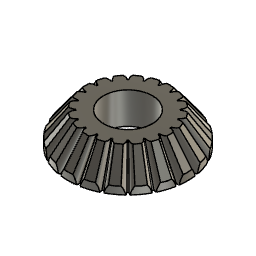
Bevel Gear (Autodesk Fusion 360 design; units mm, degrees)
Autodesk Fusion 360 part; units mm, degrees
sketch "Base" plane through (0, 0, 0) normal (0, 0, 1) x (1, 0, 0)
  line L0 (3, 40) -> (-3, 40)
  arc A0 (4.9465, 34.6487) -> (3, 40) centre (-1.791, 35.2276) ccw
  arc A1 (-3, 40) -> (-4.9465, 34.6487) centre (1.791, 35.2276) ccw
  line L1 (-9.5075, 38.9693) -> (-15.2138, 37.1152)
  arc A2 (-6.0026, 34.4814) -> (-9.5075, 38.9693) centre (-12.5893, 32.95) ccw
  arc A3 (-15.2138, 37.1152) -> (-15.4114, 31.4243) centre (-9.1826, 34.0569) ccw
  line L2 (-21.0844, 34.124) -> (-25.9385, 30.5973)
  arc A4 (-16.3642, 30.9389) -> (-21.0844, 34.124) centre (-22.1552, 27.447) ccw
  arc A5 (-25.9385, 30.5973) -> (-24.3678, 25.1239) centre (-19.2574, 29.5525) ccw
  line L3 (-30.5973, 25.9385) -> (-34.124, 21.0844)
  arc A6 (-25.1239, 24.3678) -> (-30.5973, 25.9385) centre (-29.5525, 19.2574) ccw
  arc A7 (-34.124, 21.0844) -> (-30.9389, 16.3642) centre (-27.447, 22.1552) ccw
  line L4 (-37.1152, 15.2138) -> (-38.9693, 9.5075)
  arc A8 (-31.4243, 15.4114) -> (-37.1152, 15.2138) centre (-34.0569, 9.1826) ccw
  arc A9 (-38.9693, 9.5075) -> (-34.4814, 6.0026) centre (-32.95, 12.5893) ccw
  line L5 (-40, 3) -> (-40, -3)
  arc A10 (-34.6487, 4.9465) -> (-40, 3) centre (-35.2276, -1.791) ccw
  arc A11 (-40, -3) -> (-34.6487, -4.9465) centre (-35.2276, 1.791) ccw
  line L6 (-38.9693, -9.5075) -> (-37.1152, -15.2138)
  arc A12 (-34.4814, -6.0026) -> (-38.9693, -9.5075) centre (-32.95, -12.5893) ccw
  arc A13 (-37.1152, -15.2138) -> (-31.4243, -15.4114) centre (-34.0569, -9.1826) ccw
  line L7 (-34.124, -21.0844) -> (-30.5973, -25.9385)
  arc A14 (-30.9389, -16.3642) -> (-34.124, -21.0844) centre (-27.447, -22.1552) ccw
  arc A15 (-30.5973, -25.9385) -> (-25.1239, -24.3678) centre (-29.5525, -19.2574) ccw
  line L8 (-25.9385, -30.5973) -> (-21.0844, -34.124)
  arc A16 (-24.3678, -25.1239) -> (-25.9385, -30.5973) centre (-19.2574, -29.5525) ccw
  arc A17 (-21.0844, -34.124) -> (-16.3642, -30.9389) centre (-22.1552, -27.447) ccw
  line L9 (-15.2138, -37.1152) -> (-9.5075, -38.9693)
  arc A18 (-15.4114, -31.4243) -> (-15.2138, -37.1152) centre (-9.1826, -34.0569) ccw
  arc A19 (-9.5075, -38.9693) -> (-6.0026, -34.4814) centre (-12.5893, -32.95) ccw
  line L10 (-3, -40) -> (3, -40)
  arc A20 (-4.9465, -34.6487) -> (-3, -40) centre (1.791, -35.2276) ccw
  arc A21 (3, -40) -> (4.9465, -34.6487) centre (-1.791, -35.2276) ccw
  line L11 (9.5075, -38.9693) -> (15.2138, -37.1152)
  arc A22 (6.0026, -34.4814) -> (9.5075, -38.9693) centre (12.5893, -32.95) ccw
  arc A23 (15.2138, -37.1152) -> (15.4114, -31.4243) centre (9.1826, -34.0569) ccw
  line L12 (21.0844, -34.124) -> (25.9385, -30.5973)
  arc A24 (16.3642, -30.9389) -> (21.0844, -34.124) centre (22.1552, -27.447) ccw
  arc A25 (25.9385, -30.5973) -> (24.3678, -25.1239) centre (19.2574, -29.5525) ccw
  line L13 (30.5973, -25.9385) -> (34.124, -21.0844)
  arc A26 (25.1239, -24.3678) -> (30.5973, -25.9385) centre (29.5525, -19.2574) ccw
  arc A27 (34.124, -21.0844) -> (30.9389, -16.3642) centre (27.447, -22.1552) ccw
  line L14 (37.1152, -15.2138) -> (38.9693, -9.5075)
  arc A28 (31.4243, -15.4114) -> (37.1152, -15.2138) centre (34.0569, -9.1826) ccw
  arc A29 (38.9693, -9.5075) -> (34.4814, -6.0026) centre (32.95, -12.5893) ccw
  line L15 (40, -3) -> (40, 3)
  arc A30 (34.6487, -4.9465) -> (40, -3) centre (35.2276, 1.791) ccw
  arc A31 (40, 3) -> (34.6487, 4.9465) centre (35.2276, -1.791) ccw
  line L16 (38.9693, 9.5075) -> (37.1152, 15.2138)
  arc A32 (34.4814, 6.0026) -> (38.9693, 9.5075) centre (32.95, 12.5893) ccw
  arc A33 (37.1152, 15.2138) -> (31.4243, 15.4114) centre (34.0569, 9.1826) ccw
  line L17 (34.124, 21.0844) -> (30.5973, 25.9385)
  arc A34 (30.9389, 16.3642) -> (34.124, 21.0844) centre (27.447, 22.1552) ccw
  arc A35 (30.5973, 25.9385) -> (25.1239, 24.3678) centre (29.5525, 19.2574) ccw
  line L18 (25.9385, 30.5973) -> (21.0844, 34.124)
  arc A36 (24.3678, 25.1239) -> (25.9385, 30.5973) centre (19.2574, 29.5525) ccw
  arc A37 (21.0844, 34.124) -> (16.3642, 30.9389) centre (22.1552, 27.447) ccw
  line L19 (15.2138, 37.1152) -> (9.5075, 38.9693)
  arc A38 (15.4114, 31.4243) -> (15.2138, 37.1152) centre (9.1826, 34.0569) ccw
  arc A39 (9.5075, 38.9693) -> (6.0026, 34.4814) centre (12.5893, 32.95) ccw
  arc A40 (-4.9465, 34.6487) -> (-6.0026, 34.4814) centre (0, 0) ccw
  arc A41 (-15.4114, 31.4243) -> (-16.3642, 30.9389) centre (0, 0) ccw
  arc A42 (-24.3678, 25.1239) -> (-25.1239, 24.3678) centre (0, 0) ccw
  arc A43 (-30.9389, 16.3642) -> (-31.4243, 15.4114) centre (0, 0) ccw
  arc A44 (-34.4814, 6.0026) -> (-34.6487, 4.9465) centre (0, 0) ccw
  arc A45 (-34.6487, -4.9465) -> (-34.4814, -6.0026) centre (0, 0) ccw
  arc A46 (-31.4243, -15.4114) -> (-30.9389, -16.3642) centre (0, 0) ccw
  arc A47 (-25.1239, -24.3678) -> (-24.3678, -25.1239) centre (0, 0) ccw
  arc A48 (-16.3642, -30.9389) -> (-15.4114, -31.4243) centre (0, 0) ccw
  arc A49 (-6.0026, -34.4814) -> (-4.9465, -34.6487) centre (0, 0) ccw
  arc A50 (4.9465, -34.6487) -> (6.0026, -34.4814) centre (0, 0) ccw
  arc A51 (15.4114, -31.4243) -> (16.3642, -30.9389) centre (0, 0) ccw
  arc A52 (24.3678, -25.1239) -> (25.1239, -24.3678) centre (0, 0) ccw
  arc A53 (30.9389, -16.3642) -> (31.4243, -15.4114) centre (0, 0) ccw
  arc A54 (34.4814, -6.0026) -> (34.6487, -4.9465) centre (0, 0) ccw
  arc A55 (34.6487, 4.9465) -> (34.4814, 6.0026) centre (0, 0) ccw
  arc A56 (31.4243, 15.4114) -> (30.9389, 16.3642) centre (0, 0) ccw
  arc A57 (25.1239, 24.3678) -> (24.3678, 25.1239) centre (0, 0) ccw
  arc A58 (16.3642, 30.9389) -> (15.4114, 31.4243) centre (0, 0) ccw
  arc A59 (6.0026, 34.4814) -> (4.9465, 34.6487) centre (0, 0) ccw
  line L20 (1.95, 26, 19.5) -> (-1.95, 26, 19.5)
  line L21 (6.1799, -25.3301, 19.5) -> (9.889, -24.1249, 19.5)
  line L22 (-26, 1.95, 19.5) -> (-26, -1.95, 19.5)
  line L23 (26, -1.95, 19.5) -> (26, 1.95, 19.5)
  line L24 (-16.86, -19.8883, 19.5) -> (-13.7048, -22.1806, 19.5)
  arc A60 through (-16.3305, -15.8391, 19.5) (-16.0867, -16.0867, 19.5) (-15.8391, -16.3305, 19.5)
  arc A61 through (9.889, -24.1249, 19.5) (10.3616, -22.2895, 19.5) (10.0174, -20.4258, 19.5)
  line L25 (24.1249, -9.889, 19.5) -> (25.3301, -6.1799, 19.5)
  arc A62 through (-20.4258, 10.0174, 19.5) (-22.2895, 10.3616, 19.5) (-24.1249, 9.889, 19.5)
  arc A63 through (-9.889, 24.1249, 19.5) (-10.3616, 22.2895, 19.5) (-10.0174, 20.4258, 19.5)
  line L26 (-19.8883, 16.86, 19.5) -> (-22.1806, 13.7048, 19.5)
  arc A64 through (22.5217, -3.2152, 19.5) (24.4005, -2.9666, 19.5) (26, -1.95, 19.5)
  arc A65 through (1.95, -26, 19.5) (2.9666, -24.4005, 19.5) (3.2152, -22.5217, 19.5)
  arc A66 through (3.9017, -22.4129, 19.5) (4.7188, -24.123, 19.5) (6.1799, -25.3301, 19.5)
  arc A67 through (16.3305, -15.8391, 19.5) (17.9967, -16.7423, 19.5) (19.8883, -16.86, 19.5)
  arc A68 through (-10.6367, 20.1103, 19.5) (-11.9422, 21.4841, 19.5) (-13.7048, 22.1806, 19.5)
  line L27 (-24.1249, 9.889, 19.5) -> (-25.3301, 6.1799, 19.5)
  arc A69 through (-24.1249, -9.889, 19.5) (-22.2895, -10.3616, 19.5) (-20.4258, -10.0174, 19.5)
  arc A70 through (-16.3305, 15.8391, 19.5) (-17.9967, 16.7423, 19.5) (-19.8883, 16.86, 19.5)
  arc A71 through (-26, -1.95, 19.5) (-24.4005, -2.9666, 19.5) (-22.5217, -3.2152, 19.5)
  arc A72 through (15.8391, 16.3305, 19.5) (16.7423, 17.9967, 19.5) (16.86, 19.8883, 19.5)
  arc A73 through (-20.4258, -10.0174, 19.5) (-20.2704, -10.3283, 19.5) (-20.1103, -10.6367, 19.5)
  line L28 (-9.889, -24.1249, 19.5) -> (-6.1799, -25.3301, 19.5)
  arc A74 through (24.1249, 9.889, 19.5) (22.2895, 10.3616, 19.5) (20.4258, 10.0174, 19.5)
  line L29 (-22.1806, -13.7048, 19.5) -> (-19.8883, -16.86, 19.5)
  arc A75 through (16.3305, 15.8391, 19.5) (16.0867, 16.0867, 19.5) (15.8391, 16.3305, 19.5)
  line L30 (19.8883, -16.86, 19.5) -> (22.1806, -13.7048, 19.5)
  line L31 (9.889, 24.1249, 19.5) -> (6.1799, 25.3301, 19.5)
  arc A76 through (-15.8391, -16.3305, 19.5) (-16.7423, -17.9967, 19.5) (-16.86, -19.8883, 19.5)
  arc A77 through (-15.8391, 16.3305, 19.5) (-16.0867, 16.0867, 19.5) (-16.3305, 15.8391, 19.5)
  arc A78 through (-22.5217, -3.2152, 19.5) (-22.4699, -3.5589, 19.5) (-22.4129, -3.9017, 19.5)
  arc A79 through (25.3301, -6.1799, 19.5) (24.123, -4.7188, 19.5) (22.4129, -3.9017, 19.5)
  line L32 (-13.7048, 22.1806, 19.5) -> (-16.86, 19.8883, 19.5)
  arc A80 through (22.1806, -13.7048, 19.5) (21.4841, -11.9422, 19.5) (20.1103, -10.6367, 19.5)
  arc A81 through (3.2152, -22.5217, 19.5) (3.5589, -22.4699, 19.5) (3.9017, -22.4129, 19.5)
  arc A82 through (-22.1806, 13.7048, 19.5) (-21.4841, 11.9422, 19.5) (-20.1103, 10.6367, 19.5)
  arc A83 through (22.4129, -3.9017, 19.5) (22.4699, -3.5589, 19.5) (22.5217, -3.2152, 19.5)
  arc A84 through (-10.0174, 20.4258, 19.5) (-10.3283, 20.2704, 19.5) (-10.6367, 20.1103, 19.5)
  arc A85 through (-3.2152, 22.5217, 19.5) (-3.5589, 22.4699, 19.5) (-3.9017, 22.4129, 19.5)
  arc A86 through (-1.95, 26, 19.5) (-2.9666, 24.4005, 19.5) (-3.2152, 22.5217, 19.5)
  arc A87 through (-22.4129, 3.9017, 19.5) (-22.4699, 3.5589, 19.5) (-22.5217, 3.2152, 19.5)
  arc A88 through (-16.86, 19.8883, 19.5) (-16.7423, 17.9967, 19.5) (-15.8391, 16.3305, 19.5)
  arc A89 through (-3.9017, 22.4129, 19.5) (-4.7188, 24.123, 19.5) (-6.1799, 25.3301, 19.5)
  arc A90 through (-25.3301, 6.1799, 19.5) (-24.123, 4.7188, 19.5) (-22.4129, 3.9017, 19.5)
  arc A91 through (-22.5217, 3.2152, 19.5) (-24.4005, 2.9666, 19.5) (-26, 1.95, 19.5)
  arc A92 through (-10.6367, -20.1103, 19.5) (-10.3283, -20.2704, 19.5) (-10.0174, -20.4258, 19.5)
  arc A93 through (-20.1103, 10.6367, 19.5) (-20.2704, 10.3283, 19.5) (-20.4258, 10.0174, 19.5)
  arc A94 through (-20.1103, -10.6367, 19.5) (-21.4841, -11.9422, 19.5) (-22.1806, -13.7048, 19.5)
  arc A95 through (20.1103, 10.6367, 19.5) (21.4841, 11.9422, 19.5) (22.1806, 13.7048, 19.5)
  arc A96 through (3.9017, 22.4129, 19.5) (3.5589, 22.4699, 19.5) (3.2152, 22.5217, 19.5)
  arc A97 through (22.4129, 3.9017, 19.5) (24.123, 4.7188, 19.5) (25.3301, 6.1799, 19.5)
  arc A98 through (3.2152, 22.5217, 19.5) (2.9666, 24.4005, 19.5) (1.95, 26, 19.5)
  arc A99 through (-19.8883, -16.86, 19.5) (-17.9967, -16.7423, 19.5) (-16.3305, -15.8391, 19.5)
  arc A100 through (10.0174, -20.4258, 19.5) (10.3283, -20.2704, 19.5) (10.6367, -20.1103, 19.5)
  arc A101 through (10.6367, 20.1103, 19.5) (10.3283, 20.2704, 19.5) (10.0174, 20.4258, 19.5)
  arc A102 through (15.8391, -16.3305, 19.5) (16.0867, -16.0867, 19.5) (16.3305, -15.8391, 19.5)
  arc A103 through (13.7048, 22.1806, 19.5) (11.9422, 21.4841, 19.5) (10.6367, 20.1103, 19.5)
  arc A104 through (10.6367, -20.1103, 19.5) (11.9422, -21.4841, 19.5) (13.7048, -22.1806, 19.5)
  arc A105 through (20.4258, -10.0174, 19.5) (22.2895, -10.3616, 19.5) (24.1249, -9.889, 19.5)
  arc A106 through (-3.9017, -22.4129, 19.5) (-3.5589, -22.4699, 19.5) (-3.2152, -22.5217, 19.5)
  line L33 (16.86, 19.8883, 19.5) -> (13.7048, 22.1806, 19.5)
  arc A107 through (16.86, -19.8883, 19.5) (16.7423, -17.9967, 19.5) (15.8391, -16.3305, 19.5)
  arc A108 through (26, 1.95, 19.5) (24.4005, 2.9666, 19.5) (22.5217, 3.2152, 19.5)
  line L34 (22.1806, 13.7048, 19.5) -> (19.8883, 16.86, 19.5)
  arc A109 through (6.1799, 25.3301, 19.5) (4.7188, 24.123, 19.5) (3.9017, 22.4129, 19.5)
  arc A110 through (19.8883, 16.86, 19.5) (17.9967, 16.7423, 19.5) (16.3305, 15.8391, 19.5)
  arc A111 through (-6.1799, -25.3301, 19.5) (-4.7188, -24.123, 19.5) (-3.9017, -22.4129, 19.5)
  arc A112 through (10.0174, 20.4258, 19.5) (10.3616, 22.2895, 19.5) (9.889, 24.1249, 19.5)
  arc A113 through (-10.0174, -20.4258, 19.5) (-10.3616, -22.2895, 19.5) (-9.889, -24.1249, 19.5)
  arc A114 through (-3.2152, -22.5217, 19.5) (-2.9666, -24.4005, 19.5) (-1.95, -26, 19.5)
  arc A115 through (22.5217, 3.2152, 19.5) (22.4699, 3.5589, 19.5) (22.4129, 3.9017, 19.5)
  arc A116 through (20.4258, 10.0174, 19.5) (20.2704, 10.3283, 19.5) (20.1103, 10.6367, 19.5)
  line L35 (-25.3301, -6.1799, 19.5) -> (-24.1249, -9.889, 19.5)
  line L36 (25.3301, 6.1799, 19.5) -> (24.1249, 9.889, 19.5)
  arc A117 through (20.1103, -10.6367, 19.5) (20.2704, -10.3283, 19.5) (20.4258, -10.0174, 19.5)
  arc A118 through (-22.4129, -3.9017, 19.5) (-24.123, -4.7188, 19.5) (-25.3301, -6.1799, 19.5)
  line L37 (13.7048, -22.1806, 19.5) -> (16.86, -19.8883, 19.5)
  line L38 (-1.95, -26, 19.5) -> (1.95, -26, 19.5)
  arc A119 through (-13.7048, -22.1806, 19.5) (-11.9422, -21.4841, 19.5) (-10.6367, -20.1103, 19.5)
  line L39 (-6.1799, 25.3301, 19.5) -> (-9.889, 24.1249, 19.5)
  dimension "d7" = 360
  constraint coincident A40.centre A41.centre
  constraint concentric A40 A41
  constraint concentric A41 A42
  constraint concentric A42 A43
  constraint concentric A43 A44
  constraint concentric A44 A45
  constraint concentric A45 A46
  constraint concentric A46 A47
  constraint concentric A47 A48
  constraint concentric A48 A49
  constraint concentric A49 A50
  constraint concentric A50 A51
  constraint concentric A51 A52
  constraint concentric A52 A53
  constraint concentric A53 A54
  constraint concentric A54 A55
  constraint concentric A55 A56
  constraint concentric A56 A57
  constraint concentric A57 A58
  constraint concentric A58 A59
loft "Loft1" add profiles "Base", "Base" section 1 contours L20 L21 L22 L23 L24 A60 A61 L25 A62 A63 L26 A64 A65 A66 A67 A68 L27 A69 A70 A71 A72 A73 L28 A74 L29 A75 L30 L31 A76 A77 A78 A79 L32 A80 A81 A82 A83 A84 A85 A86 A87 A88 A89 A90 A91 A92 A93 A94 A95 A96 A97 A98 A99 A100 A101 A102 A103 A104 A105 A106 L33 A107 A108 L34 A109 A110 A111 A112 A113 A114 A115 A116 L35 L36 A117 A118 L37 L38 A119 L39 in plane through (0, 0, 19.5) normal (0, 0, 1) section 2
sketch "Cut" plane through (0, 0, 0) normal (0, 0, -1) x (1, 0, 0)
  line L0 (-15.2138, -37.1152) -> (-9.5075, -38.9693)
  arc A0 (-9.5075, -38.9693) -> (-6.0026, -34.4814) centre (-12.5893, -32.95) ccw
  arc A1 (-6.0026, -34.4814) -> (-4.9465, -34.6487) centre (0, 0) ccw
  arc A2 (-4.9465, -34.6487) -> (-3, -40) centre (1.791, -35.2276) ccw
  line L1 (-3, -40) -> (3, -40)
  arc A3 (3, -40) -> (4.9465, -34.6487) centre (-1.791, -35.2276) ccw
  arc A4 (4.9465, -34.6487) -> (6.0026, -34.4814) centre (0, 0) ccw
  arc A5 (6.0026, -34.4814) -> (9.5075, -38.9693) centre (12.5893, -32.95) ccw
  line L2 (9.5075, -38.9693) -> (15.2138, -37.1152)
  arc A6 (15.2138, -37.1152) -> (15.4114, -31.4243) centre (9.1826, -34.0569) ccw
  arc A7 (15.4114, -31.4243) -> (16.3642, -30.9389) centre (0, 0) ccw
  arc A8 (16.3642, -30.9389) -> (21.0844, -34.124) centre (22.1552, -27.447) ccw
  line L3 (21.0844, -34.124) -> (25.9385, -30.5973)
  arc A9 (25.9385, -30.5973) -> (24.3678, -25.1239) centre (19.2574, -29.5525) ccw
  arc A10 (24.3678, -25.1239) -> (25.1239, -24.3678) centre (0, 0) ccw
  arc A11 (25.1239, -24.3678) -> (30.5973, -25.9385) centre (29.5525, -19.2574) ccw
  line L4 (30.5973, -25.9385) -> (34.124, -21.0844)
  arc A12 (34.124, -21.0844) -> (30.9389, -16.3642) centre (27.447, -22.1552) ccw
  arc A13 (30.9389, -16.3642) -> (31.4243, -15.4114) centre (0, 0) ccw
  arc A14 (31.4243, -15.4114) -> (37.1152, -15.2138) centre (34.0569, -9.1826) ccw
  line L5 (37.1152, -15.2138) -> (38.9693, -9.5075)
  arc A15 (38.9693, -9.5075) -> (34.4814, -6.0026) centre (32.95, -12.5893) ccw
  arc A16 (34.4814, -6.0026) -> (34.6487, -4.9465) centre (0, 0) ccw
  arc A17 (34.6487, -4.9465) -> (40, -3) centre (35.2276, 1.791) ccw
  line L6 (40, -3) -> (40, 3)
  arc A18 (40, 3) -> (34.6487, 4.9465) centre (35.2276, -1.791) ccw
  arc A19 (34.6487, 4.9465) -> (34.4814, 6.0026) centre (0, 0) ccw
  arc A20 (34.4814, 6.0026) -> (38.9693, 9.5075) centre (32.95, 12.5893) ccw
  line L7 (38.9693, 9.5075) -> (37.1152, 15.2138)
  arc A21 (37.1152, 15.2138) -> (31.4243, 15.4114) centre (34.0569, 9.1826) ccw
  arc A22 (31.4243, 15.4114) -> (30.9389, 16.3642) centre (0, 0) ccw
  arc A23 (30.9389, 16.3642) -> (34.124, 21.0844) centre (27.447, 22.1552) ccw
  line L8 (34.124, 21.0844) -> (30.5973, 25.9385)
  arc A24 (30.5973, 25.9385) -> (25.1239, 24.3678) centre (29.5525, 19.2574) ccw
  arc A25 (25.1239, 24.3678) -> (24.3678, 25.1239) centre (0, 0) ccw
  arc A26 (24.3678, 25.1239) -> (25.9385, 30.5973) centre (19.2574, 29.5525) ccw
  line L9 (25.9385, 30.5973) -> (21.0844, 34.124)
  arc A27 (21.0844, 34.124) -> (16.3642, 30.9389) centre (22.1552, 27.447) ccw
  arc A28 (16.3642, 30.9389) -> (15.4114, 31.4243) centre (0, 0) ccw
  arc A29 (15.4114, 31.4243) -> (15.2138, 37.1152) centre (9.1826, 34.0569) ccw
  line L10 (15.2138, 37.1152) -> (9.5075, 38.9693)
  arc A30 (9.5075, 38.9693) -> (6.0026, 34.4814) centre (12.5893, 32.95) ccw
  arc A31 (6.0026, 34.4814) -> (4.9465, 34.6487) centre (0, 0) ccw
  arc A32 (4.9465, 34.6487) -> (3, 40) centre (-1.791, 35.2276) ccw
  line L11 (3, 40) -> (-3, 40)
  arc A33 (-3, 40) -> (-4.9465, 34.6487) centre (1.791, 35.2276) ccw
  arc A34 (-4.9465, 34.6487) -> (-6.0026, 34.4814) centre (0, 0) ccw
  arc A35 (-6.0026, 34.4814) -> (-9.5075, 38.9693) centre (-12.5893, 32.95) ccw
  line L12 (-9.5075, 38.9693) -> (-15.2138, 37.1152)
  arc A36 (-15.2138, 37.1152) -> (-15.4114, 31.4243) centre (-9.1826, 34.0569) ccw
  arc A37 (-15.4114, 31.4243) -> (-16.3642, 30.9389) centre (0, 0) ccw
  arc A38 (-16.3642, 30.9389) -> (-21.0844, 34.124) centre (-22.1552, 27.447) ccw
  line L13 (-21.0844, 34.124) -> (-25.9385, 30.5973)
  arc A39 (-25.9385, 30.5973) -> (-24.3678, 25.1239) centre (-19.2574, 29.5525) ccw
  arc A40 (-24.3678, 25.1239) -> (-25.1239, 24.3678) centre (0, 0) ccw
  arc A41 (-25.1239, 24.3678) -> (-30.5973, 25.9385) centre (-29.5525, 19.2574) ccw
  line L14 (-30.5973, 25.9385) -> (-34.124, 21.0844)
  arc A42 (-34.124, 21.0844) -> (-30.9389, 16.3642) centre (-27.447, 22.1552) ccw
  arc A43 (-30.9389, 16.3642) -> (-31.4243, 15.4114) centre (0, 0) ccw
  arc A44 (-31.4243, 15.4114) -> (-37.1152, 15.2138) centre (-34.0569, 9.1826) ccw
  line L15 (-37.1152, 15.2138) -> (-38.9693, 9.5075)
  arc A45 (-38.9693, 9.5075) -> (-34.4814, 6.0026) centre (-32.95, 12.5893) ccw
  arc A46 (-34.4814, 6.0026) -> (-34.6487, 4.9465) centre (0, 0) ccw
  arc A47 (-34.6487, 4.9465) -> (-40, 3) centre (-35.2276, -1.791) ccw
  line L16 (-40, 3) -> (-40, -3)
  arc A48 (-40, -3) -> (-34.6487, -4.9465) centre (-35.2276, 1.791) ccw
  arc A49 (-34.6487, -4.9465) -> (-34.4814, -6.0026) centre (0, 0) ccw
  arc A50 (-34.4814, -6.0026) -> (-38.9693, -9.5075) centre (-32.95, -12.5893) ccw
  line L17 (-38.9693, -9.5075) -> (-37.1152, -15.2138)
  arc A51 (-37.1152, -15.2138) -> (-31.4243, -15.4114) centre (-34.0569, -9.1826) ccw
  arc A52 (-31.4243, -15.4114) -> (-30.9389, -16.3642) centre (0, 0) ccw
  arc A53 (-30.9389, -16.3642) -> (-34.124, -21.0844) centre (-27.447, -22.1552) ccw
  line L18 (-34.124, -21.0844) -> (-30.5973, -25.9385)
  arc A54 (-30.5973, -25.9385) -> (-25.1239, -24.3678) centre (-29.5525, -19.2574) ccw
  arc A55 (-25.1239, -24.3678) -> (-24.3678, -25.1239) centre (0, 0) ccw
  arc A56 (-24.3678, -25.1239) -> (-25.9385, -30.5973) centre (-19.2574, -29.5525) ccw
  line L19 (-25.9385, -30.5973) -> (-21.0844, -34.124)
  arc A57 (-21.0844, -34.124) -> (-16.3642, -30.9389) centre (-22.1552, -27.447) ccw
  arc A58 (-16.3642, -30.9389) -> (-15.4114, -31.4243) centre (0, 0) ccw
  arc A59 (-15.4114, -31.4243) -> (-15.2138, -37.1152) centre (-9.1826, -34.0569) ccw
  circle A60 centre (0, 0) radius 36.7638
  circle A61 centre (0, 0) radius 43.0116
  constraint concentric A1 A60
  constraint concentric A60 A61
extrude "Extrude1" cut sketch "Cut" against normal blind 10 contours L0 A0 A59 A60 | A56 L19 A57 A60 | A2 L1 A3 A60 | A53 L18 A54 A60 | A5 L2 A6 A60 | A50 L17 A51 A60 | A8 L3 A9 A60 | A47 L16 A48 A60 | A11 L4 A12 A60 | A44 L15 A45 A60 | A14 L5 A15 A60 | A41 L14 A42 A60 | A17 L6 A18 A60 | A38 L13 A39 A60 | A20 L7 A21 A60 | A35 L12 A36 A60 | A23 L8 A24 A60 | A32 L11 A33 A60 | A26 L9 A27 A60 | A29 L10 A30 A60 | A61
sketch "Hole" plane through (0, 0, 19.5) normal (0, 0, 1) x (-1, 0, 0)
  line L0 (6.1799, -25.3301) -> (9.889, -24.1249)
  arc A0 (9.889, -24.1249) -> (10.0174, -20.4258) centre (5.9687, -22.137) ccw
  arc A1 (10.0174, -20.4258) -> (10.6367, -20.1103) centre (0, 0) ccw
  arc A2 (10.6367, -20.1103) -> (13.7048, -22.1806) centre (14.4009, -17.8406) ccw
  line L1 (13.7048, -22.1806) -> (16.86, -19.8883)
  arc A3 (16.86, -19.8883) -> (15.8391, -16.3305) centre (12.5173, -19.2091) ccw
  arc A4 (15.8391, -16.3305) -> (16.3305, -15.8391) centre (0, 0) ccw
  arc A5 (16.3305, -15.8391) -> (19.8883, -16.86) centre (19.2091, -12.5173) ccw
  line L2 (19.8883, -16.86) -> (22.1806, -13.7048)
  arc A6 (22.1806, -13.7048) -> (20.1103, -10.6367) centre (17.8406, -14.4009) ccw
  arc A7 (20.1103, -10.6367) -> (20.4258, -10.0174) centre (0, 0) ccw
  arc A8 (20.4258, -10.0174) -> (24.1249, -9.889) centre (22.137, -5.9687) ccw
  line L3 (24.1249, -9.889) -> (25.3301, -6.1799)
  arc A9 (25.3301, -6.1799) -> (22.4129, -3.9017) centre (21.4175, -8.183) ccw
  arc A10 (22.4129, -3.9017) -> (22.5217, -3.2152) centre (0, 0) ccw
  arc A11 (22.5217, -3.2152) -> (26, -1.95) centre (22.898, 1.1641) ccw
  line L4 (26, -1.95) -> (26, 1.95)
  arc A12 (26, 1.95) -> (22.5217, 3.2152) centre (22.898, -1.1641) ccw
  arc A13 (22.5217, 3.2152) -> (22.4129, 3.9017) centre (0, 0) ccw
  arc A14 (22.4129, 3.9017) -> (25.3301, 6.1799) centre (21.4175, 8.183) ccw
  line L5 (25.3301, 6.1799) -> (24.1249, 9.889)
  arc A15 (24.1249, 9.889) -> (20.4258, 10.0174) centre (22.137, 5.9687) ccw
  arc A16 (20.4258, 10.0174) -> (20.1103, 10.6367) centre (0, 0) ccw
  arc A17 (20.1103, 10.6367) -> (22.1806, 13.7048) centre (17.8406, 14.4009) ccw
  line L6 (22.1806, 13.7048) -> (19.8883, 16.86)
  arc A18 (19.8883, 16.86) -> (16.3305, 15.8391) centre (19.2091, 12.5173) ccw
  arc A19 (16.3305, 15.8391) -> (15.8391, 16.3305) centre (0, 0) ccw
  arc A20 (15.8391, 16.3305) -> (16.86, 19.8883) centre (12.5173, 19.2091) ccw
  line L7 (16.86, 19.8883) -> (13.7048, 22.1806)
  arc A21 (13.7048, 22.1806) -> (10.6367, 20.1103) centre (14.4009, 17.8406) ccw
  arc A22 (10.6367, 20.1103) -> (10.0174, 20.4258) centre (0, 0) ccw
  arc A23 (10.0174, 20.4258) -> (9.889, 24.1249) centre (5.9687, 22.137) ccw
  line L8 (9.889, 24.1249) -> (6.1799, 25.3301)
  arc A24 (6.1799, 25.3301) -> (3.9017, 22.4129) centre (8.183, 21.4175) ccw
  arc A25 (3.9017, 22.4129) -> (3.2152, 22.5217) centre (0, 0) ccw
  arc A26 (3.2152, 22.5217) -> (1.95, 26) centre (-1.1641, 22.898) ccw
  line L9 (1.95, 26) -> (-1.95, 26)
  arc A27 (-1.95, 26) -> (-3.2152, 22.5217) centre (1.1641, 22.898) ccw
  arc A28 (-3.2152, 22.5217) -> (-3.9017, 22.4129) centre (0, 0) ccw
  arc A29 (-3.9017, 22.4129) -> (-6.1799, 25.3301) centre (-8.183, 21.4175) ccw
  line L10 (-6.1799, 25.3301) -> (-9.889, 24.1249)
  arc A30 (-9.889, 24.1249) -> (-10.0174, 20.4258) centre (-5.9687, 22.137) ccw
  arc A31 (-10.0174, 20.4258) -> (-10.6367, 20.1103) centre (0, 0) ccw
  arc A32 (-10.6367, 20.1103) -> (-13.7048, 22.1806) centre (-14.4009, 17.8406) ccw
  line L11 (-13.7048, 22.1806) -> (-16.86, 19.8883)
  arc A33 (-16.86, 19.8883) -> (-15.8391, 16.3305) centre (-12.5173, 19.2091) ccw
  arc A34 (-15.8391, 16.3305) -> (-16.3305, 15.8391) centre (0, 0) ccw
  arc A35 (-16.3305, 15.8391) -> (-19.8883, 16.86) centre (-19.2091, 12.5173) ccw
  line L12 (-19.8883, 16.86) -> (-22.1806, 13.7048)
  arc A36 (-22.1806, 13.7048) -> (-20.1103, 10.6367) centre (-17.8406, 14.4009) ccw
  arc A37 (-20.1103, 10.6367) -> (-20.4258, 10.0174) centre (0, 0) ccw
  arc A38 (-20.4258, 10.0174) -> (-24.1249, 9.889) centre (-22.137, 5.9687) ccw
  line L13 (-24.1249, 9.889) -> (-25.3301, 6.1799)
  arc A39 (-25.3301, 6.1799) -> (-22.4129, 3.9017) centre (-21.4175, 8.183) ccw
  arc A40 (-22.4129, 3.9017) -> (-22.5217, 3.2152) centre (0, 0) ccw
  arc A41 (-22.5217, 3.2152) -> (-26, 1.95) centre (-22.898, -1.1641) ccw
  line L14 (-26, 1.95) -> (-26, -1.95)
  arc A42 (-26, -1.95) -> (-22.5217, -3.2152) centre (-22.898, 1.1641) ccw
  arc A43 (-22.5217, -3.2152) -> (-22.4129, -3.9017) centre (0, 0) ccw
  arc A44 (-22.4129, -3.9017) -> (-25.3301, -6.1799) centre (-21.4175, -8.183) ccw
  line L15 (-25.3301, -6.1799) -> (-24.1249, -9.889)
  arc A45 (-24.1249, -9.889) -> (-20.4258, -10.0174) centre (-22.137, -5.9687) ccw
  arc A46 (-20.4258, -10.0174) -> (-20.1103, -10.6367) centre (0, 0) ccw
  arc A47 (-20.1103, -10.6367) -> (-22.1806, -13.7048) centre (-17.8406, -14.4009) ccw
  line L16 (-22.1806, -13.7048) -> (-19.8883, -16.86)
  arc A48 (-19.8883, -16.86) -> (-16.3305, -15.8391) centre (-19.2091, -12.5173) ccw
  arc A49 (-16.3305, -15.8391) -> (-15.8391, -16.3305) centre (0, 0) ccw
  arc A50 (-15.8391, -16.3305) -> (-16.86, -19.8883) centre (-12.5173, -19.2091) ccw
  line L17 (-16.86, -19.8883) -> (-13.7048, -22.1806)
  arc A51 (-13.7048, -22.1806) -> (-10.6367, -20.1103) centre (-14.4009, -17.8406) ccw
  arc A52 (-10.6367, -20.1103) -> (-10.0174, -20.4258) centre (0, 0) ccw
  arc A53 (-10.0174, -20.4258) -> (-9.889, -24.1249) centre (-5.9687, -22.137) ccw
  line L18 (-9.889, -24.1249) -> (-6.1799, -25.3301)
  arc A54 (-6.1799, -25.3301) -> (-3.9017, -22.4129) centre (-8.183, -21.4175) ccw
  arc A55 (-3.9017, -22.4129) -> (-3.2152, -22.5217) centre (0, 0) ccw
  arc A56 (-3.2152, -22.5217) -> (-1.95, -26) centre (1.1641, -22.898) ccw
  line L19 (-1.95, -26) -> (1.95, -26)
  arc A57 (1.95, -26) -> (3.2152, -22.5217) centre (-1.1641, -22.898) ccw
  arc A58 (3.2152, -22.5217) -> (3.9017, -22.4129) centre (0, 0) ccw
  arc A59 (3.9017, -22.4129) -> (6.1799, -25.3301) centre (8.183, -21.4175) ccw
  circle A60 centre (0, 0) radius 15
  dimension "d12" = 30
  constraint concentric A1 A60
  measures "d12" diameter of A60
extrude "Extrude2" cut sketch "Hole" against normal blind 55 contours A60
named bodies: "Bevel Gear"
